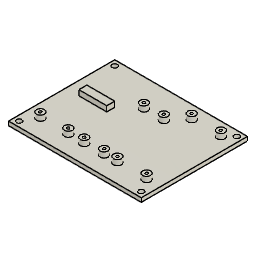
HWS Redirector mount v5 (Autodesk Fusion 360 design; units mm, degrees)
Autodesk Fusion 360 part; units mm, degrees
sketch "mount" plane through (0, 0, 0) normal (0, 0, 1) x (1, 0, 0) in component "Mount"
  line L0 (0, 0) -> (100, 0)
  line L1 (100, 0) -> (100, 80)
  line L2 (100, 80) -> (0, 80)
  line L3 (0, 80) -> (0, 0)
  line L4 (0, 14) -> (100, 14) construction
  circle A0 centre (10, 14) radius 3
  circle A1 centre (31, 14) radius 3
  circle A2 centre (43, 14) radius 3
  circle A3 centre (58, 14) radius 3
  circle A4 centre (68, 14) radius 3
  circle A5 centre (90, 14) radius 3
  line L5 (0, 59) -> (100, 59) construction
  line L6 (0, 70) -> (100, 70) construction
  line L7 (43, 14) -> (43, 59) construction
  line L8 (58, 14) -> (58, 59) construction
  line L9 (68, 14) -> (68, 70) construction
  line L10 (90, 14) -> (90, 70) construction
  circle A6 centre (43, 59) radius 3
  circle A7 centre (58, 59) radius 3
  circle A8 centre (68, 70) radius 3
  circle A9 centre (90, 70) radius 3
  circle A10 centre (4, 76) radius 2
  circle A11 centre (96, 76) radius 2
  line L11 (4, 76) -> (102.7683, 76) construction
  line L12 (96, 76) -> (96, -6.5812) construction
  line L13 (103.6465, 4) -> (-5.3628, 4) construction
  line L14 (4, 83.8921) -> (4, 81.4648) construction
  line L15 (4, 81.4648) -> (4, -6.5812) construction
  circle A12 centre (4, 4) radius 2
  circle A13 centre (96, 4) radius 2
  line L16 (10, 49) -> (31, 49)
  line L17 (31, 49) -> (31, 43)
  line L18 (31, 43) -> (10, 43)
  line L19 (10, 43) -> (10, 49)
  line L20 (10, 14) -> (10, 67.4002) construction
  circle A14 centre (10, 14) radius 1
  circle A15 centre (31, 14) radius 1
  circle A16 centre (43, 14) radius 1
  circle A17 centre (58, 14) radius 1
  circle A18 centre (68, 14) radius 1
  circle A19 centre (90, 14) radius 1
  circle A20 centre (58, 59) radius 1
  circle A21 centre (43, 59) radius 1
  circle A22 centre (68, 70) radius 1
  circle A23 centre (90, 70) radius 1
  dimension "d1" = 100
  dimension "d2" = 80
  dimension "d3" = 14
  dimension "d4" = 6
  dimension "d5" = 6
  dimension "d6" = 6
  dimension "d7" = 6
  dimension "d8" = 6
  dimension "d9" = 6
  dimension "d10" = 10
  dimension "d11" = 22
  dimension "d12" = 10
  dimension "d13" = 15
  dimension "d14" = 10
  dimension "d15" = 21
  dimension "d16" = 45
  dimension "d17" = 56
  dimension "d31" = 6
  dimension "d32" = 6
  dimension "d33" = 6
  dimension "d34" = 6
  dimension "d38" = 4
  dimension "d40" = 4
  dimension "d41" = 4
  dimension "d42" = 4
  dimension "d43" = 4
  dimension "d44" = 4
  dimension "d45" = 4
  dimension "d46" = 4
  dimension "d47" = 21
  dimension "d48" = 6
  dimension "d49" = 29
  dimension "d50" = 2
  dimension "d51" = 2
  dimension "d52" = 2
  dimension "d53" = 2
  dimension "d54" = 2
  dimension "d55" = 2
  dimension "d56" = 2
  dimension "d57" = 2
  dimension "d58" = 2
  dimension "d59" = 2
  constraint horizontal L0
  constraint vertical L1
  constraint horizontal L2
  constraint vertical L3
  constraint coincident L0.start L3.end
  constraint coincident L3 L4.start
  constraint coincident L1 L4.end
  constraint perpendicular L1 L4
  constraint coincident L4 A0.centre
  constraint coincident L4 A1.centre
  constraint coincident L4 A2.centre
  constraint coincident L4 A3.centre
  constraint coincident L4 A4.centre
  constraint coincident L4 A5.centre
  constraint coincident L3 L5.start
  constraint coincident L1 L5.end
  constraint perpendicular L1 L5
  constraint coincident L3 L6.start
  constraint coincident L1 L6.end
  constraint perpendicular L1 L6
  constraint coincident A2.centre L7.start
  constraint coincident L5 L7.end
  constraint perpendicular L5 L7
  constraint coincident A3.centre L8.start
  constraint coincident L5 L8.end
  constraint perpendicular L5 L8
  constraint coincident A4.centre L9.start
  constraint coincident L6 L9.end
  constraint perpendicular L6 L9
  constraint coincident A5.centre L10.start
  constraint coincident L6 L10.end
  constraint perpendicular L6 L10
  constraint coincident L7.end A6.centre
  constraint coincident L8.end A7.centre
  constraint coincident L9.end A8.centre
  constraint coincident L10.end A9.centre
  constraint coincident A10.centre L11.start
  constraint coincident A11.centre L12.start
  constraint perpendicular L0 L12
  constraint perpendicular L3 L13
  constraint perpendicular L2 L14
  constraint perpendicular L0 L15
  constraint horizontal L11
  constraint coincident A11.centre L11
  constraint coincident L13 A12.centre
  constraint coincident L15 A12.centre
  constraint coincident L13 A13.centre
  constraint coincident L12 A13.centre
  constraint horizontal L16
  constraint vertical L17
  constraint horizontal L18
  constraint vertical L19
  constraint coincident A0.centre L20.start
  constraint vertical L20
  constraint collinear L19 L20
  constraint concentric A0 A14
  constraint concentric A1 A15
  constraint concentric A2 A16
  constraint concentric A3 A17
  constraint concentric A4 A18
  constraint concentric A5 A19
  constraint concentric A7 A20
  constraint concentric A6 A21
  constraint concentric A8 A22
  constraint concentric A9 A23
  measures "d1" distance of L0.start L0.end
  measures "d2" distance of L0.start L2.end
  measures "d3" distance of L0 L4
  measures "d4" diameter of A0
  measures "d5" diameter of A1
  measures "d6" diameter of A2
  measures "d7" diameter of A3
  measures "d8" diameter of A4
  measures "d9" diameter of A5
  measures "d10" distance of L1 A5.centre
  measures "d11" distance of A4.centre A5.centre
  measures "d12" distance of A3.centre A4.centre
  measures "d13" distance of A2.centre A3.centre
  measures "d14" distance of L3 A0.centre
  measures "d15" distance of A0.centre A1.centre
  measures "d16" distance of L4 L5
  measures "d17" distance of L4 L6
  measures "d31" diameter of A6
  measures "d32" diameter of A7
  measures "d33" diameter of A8
  measures "d34" diameter of A9
  measures "d38" diameter of A10
  measures "d40" distance of L2 A10.centre
  measures "d41" diameter of A11
  measures "d42" distance of L0 L13
  measures "d43" distance of L3 L15
  measures "d44" distance of L1 L12
  measures "d45" diameter of A12
  measures "d46" diameter of A13
  measures "d47" distance of L16.start L16.end
  measures "d48" distance of L16.start L18.end
  measures "d49" distance of L4 L18
  measures "d50" diameter of A14
  measures "d51" diameter of A15
  measures "d52" diameter of A16
  measures "d53" diameter of A17
  measures "d54" diameter of A18
  measures "d55" diameter of A19
  measures "d56" diameter of A20
  measures "d57" diameter of A21
  measures "d58" diameter of A22
  measures "d59" diameter of A23
extrude "Extrude1" add sketch "mount" against normal blind 3 contours L0 L1 L2 L3 | A0 | A1 | A2 | A3 | A4 | A5 | A6 | A7 | A8 | A9 | L16 L17 L18 L19 in component "Mount"
extrude "Extrude2" add sketch "mount" along normal blind 4 and the other way blind 3 contours A0 | A1 | A2 | A3 | A4 | A5 | A6 | A7 | A8 | A9 | L16 L17 L18 L19 in component "Mount"
component "Mount" placed x (1, 0, 0) y (0, 1, 0) z (0, 0, 1) at (0, 0, 0)
named bodies: "HWS Mount"
